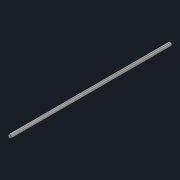
# Autodesk Inventor part: shaft1
Saved by Autodesk Inventor 2022 (Build 260153000, 153)
## iProperties
Created: 2021-10-12
Part Number: shaft1
Material: 鋼、炭素鋼
Document SubType Name: Modeling
Designer: Yuta Kage
Density: 7.85 g/cm^3
Appearance: 半つや出し
Mass: 149.895 g
Surface Area: 96.356 cm^2
Volume: 19.0949 cm^3
Description: ミスミ
Author: Yuta Kage
Autodesk Inventor part; units mm, degrees
ref_plane "YZ Plane" through (0, 0, 0) normal (1, 0, 0) x (0, 1, 0)
ref_plane "XZ Plane" through (0, 0, 0) normal (0, 1, 0) x (-1, 0, 0)
ref_plane "XY Plane" through (0, 0, 0) normal (0, 0, 1) x (1, 0, 0)
sketch "スケッチ1" plane through (0, 0, 0) normal (0, 0, 1) x (1, 0, 0)
  circle A0 centre (0, 0) radius 4
  dimension "d0" = 8
  constraints: 1 centre point, 1 coincident
  measures "d0" diameter of A0
extrude "押し出し1" add sketch "スケッチ1" along normal mid plane 400
chamfer "面取り1" distance 0.5 angle 45 2 edges at (-4, 0, 200) (-4, 0, -200)
